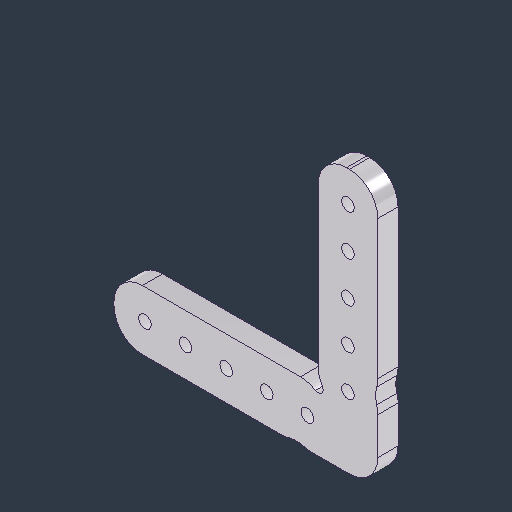
# Autodesk Inventor part: PLATE,BRACKET,ELEVATOR,STAGE1
Saved by Autodesk Inventor 2024.3 (Build 283343000, 343)
## iProperties
ILogicPurgeVersion: 0.0.0.0
OnSaveVersion: 3.4.3.0
OnSaveAssembly: COREAutomationManager
Created: 2025-01-27
Part Number: PLATE,BRACKET,ELEVATOR,STAGE1
Material: Aluminum 7075
Document SubType Name: Sheet Metal
Designer: Jthib
Density: 2.81 g/cm^3
Sheet Metal Rule: Default
Appearance: Aluminum (Polished)
Mass: 44.7906 g
Surface Area: 78.0777 cm^2
Volume: 15.9397 cm^3
Mfg Approved By: John.Thibert
Flat Pattern Width: 8.255 cm
Flat Pattern Length: 8.255 cm
Flat Pattern Area: 68.145 cm^2
Sheet Metal Width: 3.250 in
Sheet Metal Length: 3.250 in
Sheet Metal Area: 10.563 in^2
ModelCat: Uncategorized
MaterialName: Aluminum 7075
CN_MASS: 0.04
Author: Jthib
Autodesk Inventor part; units mm, degrees
ref_plane "YZ Plane" through (0, 0, 0) normal (1, 0, 0) x (0, 1, 0)
ref_plane "XZ Plane" through (0, 0, 0) normal (0, 1, 0) x (-1, 0, 0)
ref_plane "XY Plane" through (0, 0, 0) normal (0, 0, 1) x (1, 0, 0)
sketch "Sketch1" plane through (0, 0, 0) normal (0, 0, 1) x (1, 0, 0)
  line L0 (-9.3345, 9.3345) -> (-73.2155, 9.3345)
  line L1 (-73.2155, 9.3345) -> (-73.2155, -9.3345)
  line L2 (-73.2155, -9.3345) -> (9.3345, -9.3345)
  line L3 (9.3345, -9.3345) -> (9.3345, 73.2155)
  line L4 (9.3345, 73.2155) -> (-9.3345, 73.2155)
  line L5 (0, 73.2155) -> (0, 0) construction
  line L6 (0, 0) -> (-73.2155, 0) construction
  line L7 (-9.3345, 73.2155) -> (-9.3345, 9.3345)
  line L8 (-12.7, 12.7) -> (-76.581, 12.7) construction
  line L9 (-76.581, 12.7) -> (-76.581, -12.7) construction
  line L10 (-76.581, -12.7) -> (12.7, -12.7) construction
  line L11 (12.7, -12.7) -> (12.7, 76.581) construction
  line L12 (12.7, 76.581) -> (-12.7, 76.581) construction
  line L13 (-12.7, 76.581) -> (-12.7, 12.7) construction
  line L14 (9.3345, -9.3345) -> (-9.3345, 9.3345) construction
  arc A0 (-10.922, 9.3345) -> (-9.3345, 10.922) centre (-9.3345, 9.3345) ccw
  circle A1 centre (17.272, 16.0655) radius 8.636
  circle A2 centre (-16.0655, -17.272) radius 8.636
  point P0 (9.3345, 12.6631)
  point P1 (9.3345, 19.4679)
  point P2 (-19.4679, -9.3345)
  point P3 (-12.6631, -9.3345)
  dimension "d1" = 18.669
  dimension "d2" = 82.55
  dimension "d14" = 25.4
  dimension "d48" = 1.5875
  dimension "d57" = 7.9375
  dimension "d58" = 17.272
  dimension "d59" = 25.4
  constraints: 31 end point, 13 perpendicular, 3 centre point, 2 coincident, 2 midpoint, 2 point on circle, 2 point on line, 1 horizontal, 1 symmetric about line, 7 other
  measures "d1" distance of L3.end L4.end
  measures "d2" distance of L1.end L2.end
  measures "d14" distance of L11.end L12.end
  measures "d48" radius of A0
  measures "d57" distance from line of A1.centre L3
  measures "d58" diameter of A1
  measures "d59" distance from line of A1.centre L2
extrude "Plate1" add sketch "Sketch1" along normal mid plane 6.35 contours A0 L7 L4 L3 A1 L2 A2 L1 L0
sketch "Sketch3" plane through (0, 0, -3.175) normal (0, 0, -1) x (-1, 0, 0)
  line L0 (0, 0) -> (0, 73.2155) construction
  line L1 (-9.3345, 73.2155) -> (9.3345, 73.2155) construction
  line L2 (73.2155, -9.3345) -> (-9.3345, -9.3345) construction
  point P0 (0, 12.7)
  point P1 (0, 25.4)
  point P2 (0, 38.1)
  point P3 (0, 50.8)
  point P4 (0, 63.5)
  dimension "d33" = 22.0345
  dimension "d36" = 12.7
  constraints: 2 end point, 2 vertical, 1 midpoint, 1 point on line, 4 other
  measures "d33" distance from line of L2 point (0, 12.7)
  measures "d36" distance of point (0, 12.7) point (0, 25.4)
hole "Hole3" at (0, 12.7, -3.175) at (0, 25.4, -3.175) at (0, 38.1, -3.175) at (0, 50.8, -3.175) at (0, 63.5, -3.175) direction (0, 0, 1) diameter 3.9624 end through all thread size "10-32 UNF" class "2B" standard "ANSI Unified Screw Threads"
pattern_circular "Circular Pattern1" count 2 over 90 about axis through (0, 0, -10) along (0, 0, 1) of "Hole3"
fillet "Corner Round1" radius 8.89 11 edges at (-9.3345, 73.2155, 0) (9.3345, 73.2155, 0) (-9.3345, 10.922, 0) (9.3345, -9.3345, 0) (-73.2155, 9.3345, 0) (-73.2155, -9.3345, 0) (-10.922, 9.3345, 0) (-19.4679, -9.3345, 0) (-12.6631, -9.3345, 0) (9.3345, 19.4679, 0) (9.3345, 12.6631, 0)
equation "\"d32\" = Thickness"
equation "\"BendRadius\" = Thickness"
equation "\"BendReliefWidth\" = Thickness"
equation "\"BendReliefDepth\" = 0.5 * Thickness"
equation "\"CornerReliefSize\" = 4 * Thickness"
equation "\"MinimumRemnant\" = 2 * Thickness"
equation "\"TransitionRadius\" = BendRadius"
equation "\"JacobiRadiusSize\" = BendRadius"
equation "\"GapSize\" = Thickness"
equation "\"Thickness\" = 6.35"
body "Solid1"
